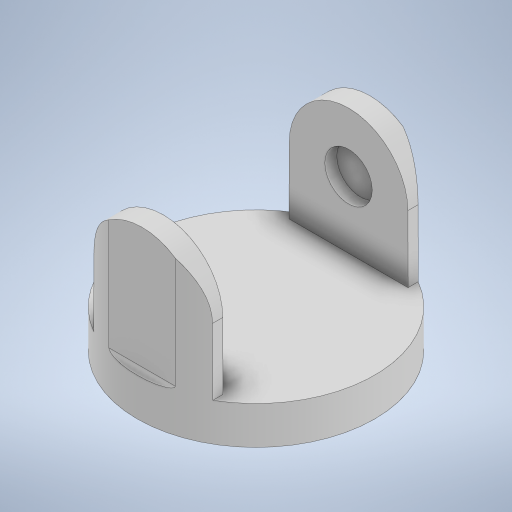
# Autodesk Inventor part: Arm 1 v0.1
Saved by Autodesk Inventor 2023 (Build 270158000, 158)
## iProperties
Created: 2024-06-24
Part Number: Arm 1 v0.1
Material: Generic
Document SubType Name: Modeling
Designer: Swoby
Density: 1 g/cm^3
Appearance: Default
Author: Swoby
Autodesk Inventor part; units mm, degrees
ref_plane "YZ Plane" through (0, 0, 0) normal (1, 0, 0) x (0, 1, 0)
ref_plane "XZ Plane" through (0, 0, 0) normal (0, 1, 0) x (-1, 0, 0)
ref_plane "XY Plane" through (0, 0, 0) normal (0, 0, 1) x (1, 0, 0)
sketch "Sketch1" plane through (0, 0, 0) normal (0, 0, 1) x (1, 0, 0)
  line L0 (0, 0) -> (47.25, 0)
  line L1 (47.25, 0) -> (47.25, -4)
  line L2 (47.25, -4) -> (50, -4)
  line L3 (50, -4) -> (50, 65)
  line L4 (50, 65) -> (0, 65)
  line L5 (0, 65) -> (0, 0)
  dimension "d0" = 100
  dimension "d1" = 94.5
  dimension "d2" = 4
  dimension "d3" = 65
  constraints: 12 end point, 4 perpendicular, 1 horizontal
  measures "d0" diameter of L3 L5
  measures "d1" diameter of L1 L5
  measures "d2" distance of L0.end L1.end
  measures "d3" distance between parallel lines of L0 L4
revolve "Revolution1" add sketch "Sketch1" angle 360 about axis through (0, 65, 0) along (0, -1, 0)
sketch "Sketch2" plane through (0, 0, 0) normal (0, 0, 1) x (1, 0, 0)
  line L0 (-50, 65) -> (-50, -4) projected
  line L1 (-50, 12) -> (50, 12)
  circle A0 centre (0, 40) radius 25
  line L2 (-50, 65) -> (50, 65) projected
  line L3 (0, 0) -> (0, 65) construction
  arc A1 (-50, 12) -> (-24.9999, 40.0686) centre (-53.3441, 40.1463) ccw
  arc A2 (24.9999, 40.0686) -> (50, 12) centre (53.3441, 40.1463) ccw
  line L4 (50, 65) -> (50, -4) projected
  point P0 (0, 12)
  point P1 (0, 65)
  dimension "d5" = 12
  dimension "d6" = 50
  dimension "d7" = 28.0686
  dimension "d8" = 28.0686
  constraints: 6 point on circle, 4 end point, 3 centre point, 3 point on line, 3 tangent, 2 midpoint, 1 perpendicular
  measures "d5" distance of L3.start point (0, 12)
  measures "d6" diameter of A0
  measures "d7" distance from line of L1 A0.start
  measures "d8" distance from line of L1 A0.end
extrude "Extrusion1" cut sketch "Sketch2" along normal through all both and the other way through all contours L2 A0 A1 L0 | L2 L4 A2 A0
sketch "Sketch4" plane through (0, 0, 0) normal (1, 0, 0) x (0, 1, 0)
  line L0 (65, 50) -> (-4, 50) projected
  line L1 (12, 50) -> (12, 50)
  line L2 (14, -48) -> (65, -48)
  line L3 (14, 48) -> (65, 48)
  line L4 (65, 50) -> (65, -50) projected
  line L5 (0, 47.25) -> (0, -47.25) projected
  line L6 (65, -50) -> (-4, -50) projected
  arc A0 (12, 50) -> (14, 48) centre (14, 50) ccw
  line L7 (12, -50) -> (12, -50)
  arc A1 (14, -48) -> (12, -50) centre (14, -50) ccw
  line L8 (65, -39) -> (12, -39)
  line L9 (12, -39) -> (12, 39)
  line L10 (12, 39) -> (65, 39)
  line L11 (65, 39) -> (65, -39)
  line L12 (12, -50) -> (65, -50)
  line L13 (65, -48) -> (65, -50)
  line L14 (12, 50) -> (65, 50)
  line L15 (65, 50) -> (65, 48)
  point P0 (0, 0)
  point P1 (12, -48)
  point P2 (65, 39)
  dimension "d14" = 2
  dimension "d15" = 12
  dimension "d16" = 2
  dimension "d17" = 2
  dimension "d18" = 2
  dimension "d19" = 12
  dimension "d20" = 9
  dimension "d21" = 9
  constraints: 24 end point, 8 point on line, 4 parallel, 4 point on circle, 4 tangent, 2 centre point, 2 horizontal, 2 perpendicular, 1 vertical
  measures "d14" distance between parallel lines of L0 L3
  measures "d15" distance between parallel lines of L5 L1
  measures "d16" distance from line of L4.end L2
  measures "d17" radius of A0
  measures "d18" radius of A1
  measures "d19" distance between parallel lines of L9 L5
  measures "d20" distance between parallel lines of L10 L3
  measures "d21" distance between parallel lines of L2 L8
extrude "Extrusion2" cut sketch "Sketch4" along normal through all both and the other way through all
sketch "Sketch5" plane through (0, 40, 48) normal (0, 0, 1) x (1, 0, 0)
  line L0 (-31.289, -28) -> (31.289, -28) projected
  line L1 (-31.289, -28) -> (-25.0769, -28)
  spline S0 degree 7 poles (-24.9999, 0.0686) (-25.0047, -1.665) (-25.1331, -3.4008) (-25.3859, -5.1281) (-25.7625, -6.8362) (-26.2611, -8.5141) (-26.8789, -10.1513) (-27.8149, -12.1783) (-28.0274, -12.6153) (-28.2486, -13.0478) (-28.478, -13.4752) (-28.7156, -13.8974) (-28.961, -14.3139) (-29.4863, -15.1662) (-29.7674, -15.6012) (-30.057, -16.029) (-30.3544, -16.4489) (-30.6593, -16.8605) (-30.971, -17.2634) (-31.289, -17.6573) knots 0 0 0 0 0 0 0 0 0.63383 0.63383 0.63383 0.63383 0.63383 0.63383 0.810222 0.810222 0.810222 0.810222 0.810222 0.810222 1 1 1 1 1 1 1 1 projected
  line L2 (-31.289, -17.6573) -> (-31.289, -28) projected
  spline S1 degree 7 poles (31.289, -17.6573) (30.9729, -17.2657) (30.6629, -16.8652) (30.3597, -16.456) (30.0639, -16.0387) (29.7758, -15.6136) (29.4961, -15.1814) (28.9731, -14.3341) (28.7285, -13.9199) (28.4918, -13.5001) (28.263, -13.075) (28.0425, -12.645) (27.8305, -12.2104) (26.8905, -10.182) (26.269, -8.5404) (25.7672, -6.8576) (25.3883, -5.1443) (25.1339, -3.4117) (25.0047, -1.6704) (24.9999, 0.0686) knots 0 0 0 0 0 0 0 0 0.188676 0.188676 0.188676 0.188676 0.188676 0.188676 0.364186 0.364186 0.364186 0.364186 0.364186 0.364186 1 1 1 1 1 1 1 1 projected
  line L3 (31.289, -28) -> (31.289, -17.6573) projected
  arc A0 (24.9999, 0.0686) -> (31.289, -17.6573) centre (53.3441, 0.1463) ccw projected
  line L4 (24.9999, 0.0686) -> (25.0769, -28)
  line L5 (25.0769, -28) -> (31.289, -28)
  arc A1 (-31.289, -17.6573) -> (-24.9999, 0.0686) centre (-53.3441, 0.1463) ccw projected
  line L6 (-24.9999, 0.0686) -> (-25.0769, -28)
  point P0 (0, -40)
  point P1 (24.9999, -28)
  constraints: 8 end point, 3 point on line, 2 tangent, 1 collinear, 2 other
extrude "Extrusion3" cut sketch "Sketch5" along normal through all both and the other way through all
sketch "Sketch6" plane through (0, 40, -39) normal (0, 0, 1) x (1, 0, 0)
  arc A0 (14, 20.7123) -> (-14, 20.7123) centre (0, 0) ccw projected
  circle A1 centre (0, 0) radius 10
  point P0 (0, -40)
  dimension "d26" = 20
  constraints: 1 centre point, 1 coincident, 2 other
  measures "d26" diameter of A1
extrude "Extrusion4" cut sketch "Sketch6" along normal blind 83 and the other way blind 5
equation "\"d8\" = d7"
equation "\"d21\" = d20"
body "Solid1"
